Autodesk Fusion 360 part; units mm, degrees
(part 2 of 4)
  arc A354 (22.3833, -33.1693) -> (21.8833, -32.6693) centre (22.3833, -32.6693) cw
  arc A355 (35.3833, -19.1693) -> (35.8833, -19.6693) centre (35.3833, -19.6693) cw
  line L355 (21.8833, -32.6693) -> (21.8833, -19.6693)
  line L356 (35.8833, -0.6193) -> (35.8833, -13.6193)
  line L357 (21.8833, -13.6193) -> (21.8833, -0.6193)
  arc A356 (35.3833, -0.1193) -> (35.8833, -0.6193) centre (35.3833, -0.6193) cw
  arc A357 (35.8833, -13.6193) -> (35.3833, -14.1193) centre (35.3833, -13.6193) cw
  line L358 (22.3833, -0.1193) -> (35.3833, -0.1193)
  arc A358 (22.3833, -14.1193) -> (21.8833, -13.6193) centre (22.3833, -13.6193) cw
  line L359 (35.3833, -14.1193) -> (22.3833, -14.1193)
  arc A359 (21.8833, -0.6193) -> (22.3833, -0.1193) centre (22.3833, -0.6193) cw
  line L360 (22.3833, 18.9307) -> (35.3833, 18.9307)
  line L361 (35.3833, 4.9307) -> (22.3833, 4.9307)
  arc A360 (21.8833, 18.4307) -> (22.3833, 18.9307) centre (22.3833, 18.4307) cw
  arc A361 (35.8833, 5.4307) -> (35.3833, 4.9307) centre (35.3833, 5.4307) cw
  line L362 (21.8833, 5.4307) -> (21.8833, 18.4307)
  arc A362 (22.3833, 4.9307) -> (21.8833, 5.4307) centre (22.3833, 5.4307) cw
  arc A363 (35.3833, 18.9307) -> (35.8833, 18.4307) centre (35.3833, 18.4307) cw
  line L363 (35.8833, 18.4307) -> (35.8833, 5.4307)
  arc A364 (22.3833, 23.9807) -> (21.8833, 24.4807) centre (22.3833, 24.4807) cw
  arc A365 (35.3833, 37.9807) -> (35.8833, 37.4807) centre (35.3833, 37.4807) cw
  line L364 (35.8833, 37.4807) -> (35.8833, 24.4807)
  arc A366 (35.8833, 24.4807) -> (35.3833, 23.9807) centre (35.3833, 24.4807) cw
  line L365 (22.3833, 37.9807) -> (35.3833, 37.9807)
  arc A367 (21.8833, 37.4807) -> (22.3833, 37.9807) centre (22.3833, 37.4807) cw
  line L366 (35.3833, 23.9807) -> (22.3833, 23.9807)
  line L367 (21.8833, 24.4807) -> (21.8833, 37.4807)
  arc A368 (21.8833, 56.5307) -> (22.3833, 57.0307) centre (22.3833, 56.5307) cw
  arc A369 (22.3833, 43.0307) -> (21.8833, 43.5307) centre (22.3833, 43.5307) cw
  line L368 (22.3833, 57.0307) -> (35.3833, 57.0307)
  line L369 (35.3833, 43.0307) -> (22.3833, 43.0307)
  line L370 (21.8833, 43.5307) -> (21.8833, 56.5307)
  arc A370 (35.8833, 43.5307) -> (35.3833, 43.0307) centre (35.3833, 43.5307) cw
  arc A371 (35.3833, 57.0307) -> (35.8833, 56.5307) centre (35.3833, 56.5307) cw
  line L371 (35.8833, 56.5307) -> (35.8833, 43.5307)
  line L372 (22.3833, 76.0807) -> (35.3833, 76.0807)
  arc A372 (35.3833, 76.0807) -> (35.8833, 75.5807) centre (35.3833, 75.5807) cw
  arc A373 (35.8833, 62.5807) -> (35.3833, 62.0807) centre (35.3833, 62.5807) cw
  arc A374 (21.8833, 75.5807) -> (22.3833, 76.0807) centre (22.3833, 75.5807) cw
  line L373 (21.8833, 62.5807) -> (21.8833, 75.5807)
  line L374 (35.8833, 75.5807) -> (35.8833, 62.5807)
  line L375 (35.3833, 62.0807) -> (22.3833, 62.0807)
  arc A375 (22.3833, 62.0807) -> (21.8833, 62.5807) centre (22.3833, 62.5807) cw
  line L376 (22.3833, 95.1307) -> (35.3833, 95.1307)
  arc A376 (35.3833, 95.1307) -> (35.8833, 94.6307) centre (35.3833, 94.6307) cw
  line L377 (35.3833, 81.1307) -> (22.3833, 81.1307)
  line L378 (35.8833, 94.6307) -> (35.8833, 81.6307)
  arc A377 (35.8833, 81.6307) -> (35.3833, 81.1307) centre (35.3833, 81.6307) cw
  line L379 (21.8833, 81.6307) -> (21.8833, 94.6307)
  arc A378 (21.8833, 94.6307) -> (22.3833, 95.1307) centre (22.3833, 94.6307) cw
  arc A379 (22.3833, 81.1307) -> (21.8833, 81.6307) centre (22.3833, 81.6307) cw
  line L380 (35.3833, 116.8495) -> (22.3833, 116.8495)
  arc A380 (22.3833, 116.8495) -> (21.8833, 117.3495) centre (22.3833, 117.3495) cw
  arc A381 (35.8833, 117.3495) -> (35.3833, 116.8495) centre (35.3833, 117.3495) cw
  arc A382 (35.3833, 130.8495) -> (35.8833, 130.3495) centre (35.3833, 130.3495) cw
  line L381 (21.8833, 117.3495) -> (21.8833, 130.3495)
  arc A383 (21.8833, 130.3495) -> (22.3833, 130.8495) centre (22.3833, 130.3495) cw
  line L382 (35.8833, 130.3495) -> (35.8833, 117.3495)
  line L383 (22.3833, 130.8495) -> (35.3833, 130.8495)
  arc A384 (19.8833, 114.9115) -> (20.3833, 115.4115) centre (20.3833, 114.9115) cw
  arc A385 (34.8833, 108.9115) -> (34.3833, 108.4115) centre (34.3833, 108.9115) cw
  line L384 (20.3833, 115.4115) -> (34.3833, 115.4115)
  line L385 (34.3833, 108.4115) -> (20.3833, 108.4115)
  line L386 (34.8833, 114.9115) -> (34.8833, 108.9115)
  arc A386 (34.3833, 115.4115) -> (34.8833, 114.9115) centre (34.3833, 114.9115) cw
  line L387 (19.8833, 108.9115) -> (19.8833, 114.9115)
  arc A387 (20.3833, 108.4115) -> (19.8833, 108.9115) centre (20.3833, 108.9115) cw
  line L388 (19.8833, 132.7875) -> (19.8833, 138.7875)
  arc A388 (34.3833, 139.2875) -> (34.8833, 138.7875) centre (34.3833, 138.7875) cw
  line L389 (20.3833, 139.2875) -> (34.3833, 139.2875)
  line L390 (34.3833, 132.2875) -> (20.3833, 132.2875)
  line L391 (34.8833, 138.7875) -> (34.8833, 132.7875)
  arc A389 (19.8833, 138.7875) -> (20.3833, 139.2875) centre (20.3833, 138.7875) cw
  arc A390 (34.8833, 132.7875) -> (34.3833, 132.2875) centre (34.3833, 132.7875) cw
  arc A391 (20.3833, 132.2875) -> (19.8833, 132.7875) centre (20.3833, 132.7875) cw
  line L392 (35.8833, 194.6432) -> (35.8833, 181.6432)
  line L393 (22.3833, 195.1432) -> (35.3833, 195.1432)
  line L394 (35.3833, 181.1432) -> (22.3833, 181.1432)
  line L395 (21.8833, 181.6432) -> (21.8833, 194.6432)
  arc A392 (35.8833, 181.6432) -> (35.3833, 181.1432) centre (35.3833, 181.6432) cw
  arc A393 (35.3833, 195.1432) -> (35.8833, 194.6432) centre (35.3833, 194.6432) cw
  arc A394 (22.3833, 181.1432) -> (21.8833, 181.6432) centre (22.3833, 181.6432) cw
  arc A395 (21.8833, 194.6432) -> (22.3833, 195.1432) centre (22.3833, 194.6432) cw
  arc A396 (41.4333, -204.6193) -> (40.9332, -204.1193) centre (41.4333, -204.1193) cw
  line L396 (54.9333, -191.1193) -> (54.9332, -204.1193)
  line L397 (40.9332, -204.1193) -> (40.9333, -191.1193)
  arc A397 (40.9333, -191.1193) -> (41.4333, -190.6193) centre (41.4333, -191.1193) cw
  line L398 (41.4333, -190.6193) -> (54.4333, -190.6193)
  arc A398 (54.9332, -204.1193) -> (54.4332, -204.6193) centre (54.4333, -204.1193) cw
  line L399 (54.4332, -204.6193) -> (41.4333, -204.6193)
  arc A399 (54.4333, -190.6193) -> (54.9332, -191.1193) centre (54.4333, -191.1193) cw
  line L400 (41.4333, -162.0443) -> (54.4333, -162.0443)
  line L401 (54.9333, -162.5443) -> (54.9332, -175.5443)
  arc A400 (41.4333, -176.0443) -> (40.9333, -175.5443) centre (41.4333, -175.5443) cw
  arc A401 (54.9332, -175.5443) -> (54.4333, -176.0443) centre (54.4333, -175.5443) cw
  arc A402 (40.9333, -162.5443) -> (41.4333, -162.0443) centre (41.4333, -162.5443) cw
  line L402 (40.9333, -175.5443) -> (40.9333, -162.5443)
  arc A403 (54.4333, -162.0443) -> (54.9333, -162.5443) centre (54.4333, -162.5443) cw
  line L403 (54.4333, -176.0443) -> (41.4333, -176.0443)
  arc A404 (54.9333, -125.538) -> (54.4333, -126.038) centre (54.4333, -125.538) cw
  line L404 (41.4333, -112.038) -> (54.4333, -112.038)
  arc A405 (41.4333, -126.038) -> (40.9333, -125.538) centre (41.4333, -125.538) cw
  line L405 (54.4333, -126.038) -> (41.4333, -126.038)
  arc A406 (40.9333, -112.538) -> (41.4333, -112.038) centre (41.4333, -112.538) cw
  arc A407 (54.4333, -112.038) -> (54.9333, -112.538) centre (54.4333, -112.538) cw
  line L406 (54.9333, -112.538) -> (54.9333, -125.538)
  line L407 (40.9333, -125.538) -> (40.9333, -112.538)
  arc A408 (54.4333, -88.2255) -> (54.9333, -88.7255) centre (54.4333, -88.7255) cw
  arc A409 (41.4333, -102.2255) -> (40.9333, -101.7255) centre (41.4333, -101.7255) cw
  arc A410 (54.9333, -101.7255) -> (54.4333, -102.2255) centre (54.4333, -101.7255) cw
  line L408 (41.4333, -88.2255) -> (54.4333, -88.2255)
  arc A411 (40.9333, -88.7255) -> (41.4333, -88.2255) centre (41.4333, -88.7255) cw
  line L409 (54.9333, -88.7255) -> (54.9333, -101.7255)
  line L410 (40.9333, -101.7255) -> (40.9333, -88.7255)
  line L411 (54.4333, -102.2255) -> (41.4333, -102.2255)
  line L412 (54.9333, -64.913) -> (54.9333, -77.913)
  arc A412 (40.9333, -64.913) -> (41.4333, -64.413) centre (41.4333, -64.913) cw
  line L413 (41.4333, -64.413) -> (54.4333, -64.413)
  line L414 (40.9333, -77.913) -> (40.9333, -64.913)
  arc A413 (54.4333, -64.413) -> (54.9333, -64.913) centre (54.4333, -64.913) cw
  arc A414 (54.9333, -77.913) -> (54.4333, -78.413) centre (54.4333, -77.913) cw
  line L415 (54.4333, -78.413) -> (41.4333, -78.413)
  arc A415 (41.4333, -78.413) -> (40.9333, -77.913) centre (41.4333, -77.913) cw
  arc A416 (40.9333, 6.5245) -> (41.4333, 7.0245) centre (41.4333, 6.5245) cw
  line L416 (40.9333, -6.4755) -> (40.9333, 6.5245)
  line L417 (54.9333, 6.5245) -> (54.9333, -6.4755)
  arc A417 (54.4333, 7.0245) -> (54.9333, 6.5245) centre (54.4333, 6.5245) cw
  arc A418 (54.9333, -6.4755) -> (54.4333, -6.9755) centre (54.4333, -6.4755) cw
  arc A419 (41.4333, -6.9755) -> (40.9333, -6.4755) centre (41.4333, -6.4755) cw
  line L418 (41.4333, 7.0245) -> (54.4333, 7.0245)
  line L419 (54.4333, -6.9755) -> (41.4333, -6.9755)
  arc A420 (53.4333, -46.4755) -> (53.9333, -46.9755) centre (53.4333, -46.9755) cw
  line L420 (39.4333, -46.4755) -> (53.4333, -46.4755)
  arc A421 (39.4333, -53.4755) -> (38.9333, -52.9755) centre (39.4333, -52.9755) cw
  arc A422 (38.9332, -46.9755) -> (39.4333, -46.4755) centre (39.4333, -46.9755) cw
  line L421 (53.9333, -46.9755) -> (53.9333, -52.9755)
  arc A423 (53.9333, -52.9755) -> (53.4333, -53.4755) centre (53.4333, -52.9755) cw
  line L422 (53.4333, -53.4755) -> (39.4333, -53.4755)
  line L423 (38.9333, -52.9755) -> (38.9332, -46.9755)
  line L424 (38.9333, 47.0245) -> (38.9333, 53.0245)
  line L425 (53.4333, 46.5245) -> (39.4333, 46.5245)
  line L426 (39.4333, 53.5245) -> (53.4333, 53.5245)
  arc A424 (39.4333, 46.5245) -> (38.9333, 47.0245) centre (39.4333, 47.0245) cw
  arc A425 (53.4333, 53.5245) -> (53.9333, 53.0245) centre (53.4333, 53.0245) cw
  line L427 (53.9333, 53.0245) -> (53.9333, 47.0245)
  arc A426 (38.9333, 53.0245) -> (39.4333, 53.5245) centre (39.4333, 53.0245) cw
  arc A427 (53.9333, 47.0245) -> (53.4333, 46.5245) centre (53.4333, 47.0245) cw
  arc A428 (40.9333, 77.962) -> (41.4333, 78.462) centre (41.4333, 77.962) cw
  arc A429 (54.9333, 64.962) -> (54.4333, 64.462) centre (54.4333, 64.962) cw
  arc A430 (54.4333, 78.462) -> (54.9333, 77.962) centre (54.4333, 77.962) cw
  line L428 (40.9333, 64.962) -> (40.9333, 77.962)
  arc A431 (41.4333, 64.462) -> (40.9333, 64.962) centre (41.4333, 64.962) cw
  line L429 (54.4333, 64.462) -> (41.4333, 64.462)
  line L430 (54.9333, 77.962) -> (54.9333, 64.962)
  line L431 (41.4333, 78.462) -> (54.4333, 78.462)
  arc A432 (40.9333, 101.7745) -> (41.4333, 102.2745) centre (41.4333, 101.7745) cw
  line L432 (54.9333, 101.7745) -> (54.9333, 88.7745)
  arc A433 (54.4333, 102.2745) -> (54.9333, 101.7745) centre (54.4333, 101.7745) cw
  arc A434 (41.4333, 88.2745) -> (40.9333, 88.7745) centre (41.4333, 88.7745) cw
  line L433 (54.4333, 88.2745) -> (41.4333, 88.2745)
  line L434 (40.9333, 88.7745) -> (40.9333, 101.7745)
  line L435 (41.4333, 102.2745) -> (54.4333, 102.2745)
  arc A435 (54.9333, 88.7745) -> (54.4333, 88.2745) centre (54.4333, 88.7745) cw
  arc A436 (54.9333, 112.587) -> (54.4333, 112.087) centre (54.4333, 112.587) cw
  arc A437 (40.9332, 125.587) -> (41.4333, 126.087) centre (41.4333, 125.587) cw
  line L436 (54.4333, 112.087) -> (41.4333, 112.087)
  arc A438 (41.4333, 112.087) -> (40.9333, 112.587) centre (41.4333, 112.587) cw
  line L437 (40.9333, 112.587) -> (40.9332, 125.587)
  line L438 (41.4333, 126.087) -> (54.4333, 126.087)
  line L439 (54.9333, 125.587) -> (54.9333, 112.587)
  arc A439 (54.4333, 126.087) -> (54.9333, 125.587) centre (54.4333, 125.587) cw
  line L440 (54.9333, 147.0182) -> (54.9333, 134.0182)
  line L441 (41.4333, 147.5182) -> (54.4333, 147.5182)
  arc A440 (40.9333, 147.0182) -> (41.4333, 147.5182) centre (41.4333, 147.0182) cw
  arc A441 (54.9333, 134.0182) -> (54.4333, 133.5182) centre (54.4333, 134.0182) cw
  line L442 (40.9333, 134.0182) -> (40.9333, 147.0182)
  arc A442 (41.4333, 133.5182) -> (40.9333, 134.0182) centre (41.4333, 134.0182) cw
  line L443 (54.4333, 133.5182) -> (41.4333, 133.5182)
  arc A443 (54.4333, 147.5182) -> (54.9333, 147.0182) centre (54.4333, 147.0182) cw
  line L444 (41.4333, 176.0932) -> (54.4333, 176.0932)
  arc A444 (54.9333, 162.5932) -> (54.4333, 162.0932) centre (54.4333, 162.5932) cw
  line L445 (40.9333, 162.5932) -> (40.9333, 175.5932)
  arc A445 (41.4333, 162.0932) -> (40.9333, 162.5932) centre (41.4333, 162.5932) cw
  line L446 (54.4333, 162.0932) -> (41.4333, 162.0932)
  arc A446 (54.4333, 176.0932) -> (54.9333, 175.5932) centre (54.4333, 175.5932) cw
  line L447 (54.9333, 175.5932) -> (54.9333, 162.5932)
  arc A447 (40.9333, 175.5932) -> (41.4333, 176.0932) centre (41.4333, 175.5932) cw
  line L448 (41.4333, 195.1432) -> (54.4333, 195.1432)
  arc A448 (54.9333, 181.6432) -> (54.4333, 181.1432) centre (54.4333, 181.6432) cw
  line L449 (40.9333, 181.6432) -> (40.9333, 194.6432)
  line L450 (54.9333, 194.6432) -> (54.9333, 181.6432)
  arc A449 (41.4333, 181.1432) -> (40.9333, 181.6432) centre (41.4333, 181.6432) cw
  arc A450 (54.4333, 195.1432) -> (54.9333, 194.6432) centre (54.4333, 194.6432) cw
  line L451 (54.4333, 181.1432) -> (41.4333, 181.1432)
  arc A451 (40.9333, 194.6432) -> (41.4333, 195.1432) centre (41.4333, 194.6432) cw
  line L452 (40.9333, 200.6932) -> (40.9333, 213.6932)
  arc A452 (54.4333, 214.1932) -> (54.9333, 213.6932) centre (54.4333, 213.6932) cw
  arc A453 (41.4333, 200.1932) -> (40.9333, 200.6932) centre (41.4333, 200.6932) cw
  line L453 (41.4333, 214.1932) -> (54.4333, 214.1932)
  line L454 (54.9333, 213.6932) -> (54.9333, 200.6932)
  arc A454 (40.9333, 213.6932) -> (41.4333, 214.1932) centre (41.4333, 213.6932) cw
  line L455 (54.4333, 200.1932) -> (41.4333, 200.1932)
  arc A455 (54.9333, 200.6932) -> (54.4333, 200.1932) centre (54.4333, 200.6932) cw
  line L456 (58.3332, -216.6443) -> (58.3333, 224.1932)
  line L457 (-61.771, -216.6443) -> (-61.771, 224.1932)
  line L458 (58.3332, -216.6443) -> (-61.771, -216.6443)
  line L459 (58.3333, 224.1932) -> (-61.771, 224.1932)
  line L460 (58.3332, -216.6443) -> (-37.7668, -216.6443)
  line L461 (-37.7668, -216.6443) -> (-37.7667, -166.6443)
  line L462 (-37.7667, -166.6443) -> (-61.771, -166.6443)
  line L463 (-61.771, 150.0182) -> (-28.2417, 150.0182)
  line L464 (-28.2417, 150.0182) -> (-28.2417, 224.1932)
  line L465 (-28.2417, 224.1932) -> (58.3333, 224.1932)
  line L466 (-61.771, 150.0182) -> (-61.771, -166.6443) construction
  line L467 (63.4708, 230.5) -> (-67.5292, 230.5)
  line L468 (-67.5292, 230.5) -> (-67.5292, -230.5)
  line L469 (-67.5292, -230.5) -> (63.4708, -230.5)
  line L470 (63.4708, -230.5) -> (63.4708, 230.5)
  line L471 (-67.0292, -230) -> (62.9708, -230)
  line L472 (-66.7431, 215) -> (-32.0292, 215)
  line L473 (-66.7431, 150) -> (-66.7431, -166.6443)
  line L474 (-66.7431, -166.6443) -> (-37.7667, -166.6443)
  line L475 (-37.7667, -166.6443) -> (-37.7668, -230)
  line L476 (-66.7431, 230) -> (-66.7431, 215)
  line L477 (-37.7668, -230) -> (62.9708, -230)
  line L478 (62.9708, 230) -> (-66.7431, 230)
  line L479 (-32.0292, 215) -> (-32.0292, 150)
  line L480 (-32.0292, 150) -> (-66.7431, 150)
  line L481 (62.9708, -230) -> (62.9708, 230)
  line L482 (-66.7431, 150) -> (-66.7431, 230)
  line L483 (-66.7431, 230) -> (62.9708, 230)
  line L484 (62.9708, 230) -> (62.9708, 231.4)
  line L485 (62.9708, 231.4) -> (-66.7431, 231.4)
  line L486 (-66.7431, 231.4) -> (-66.7431, 230)
  line L487 (-37.7668, -230) -> (62.9708, -230)
  line L488 (62.9708, -230) -> (62.9708, -228.6)
  line L489 (62.9708, -228.6) -> (-37.7668, -228.6)
  line L490 (-37.7668, -228.6) -> (-37.7668, -230)
  line L491 (62.9708, -230) -> (61.7708, -230)
  line L492 (61.7708, -230) -> (61.7708, 231.4118)
  line L493 (61.7708, 231.4118) -> (62.9708, 231.4118)
  line L494 (62.9708, 231.4118) -> (62.9708, -230)
  line L495 (-66.7431, -166.6443) -> (-67.9431, -166.6443)
  line L496 (-67.9431, -166.6443) -> (-67.9431, 231.4)
  line L497 (-67.9431, 231.4) -> (-66.7431, 231.4)
  line L498 (-66.7431, 231.4) -> (-66.7431, -166.6443)
  line L499 (-67.9431, -166.6443) -> (-62.9431, -166.6443) construction
  line L500 (-62.9431, -166.6443) -> (-62.9431, -161.6443) construction
  line L501 (-62.9431, -161.6443) -> (-67.9431, -161.6443) construction
  line L502 (-67.9431, -161.6443) -> (-67.9431, -166.6443) construction
  circle A456 centre (-62.9431, -161.6443) radius 1.5
  line L503 (-62.9431, -161.6443) -> (-42.9431, -161.6443) construction
  circle A457 centre (-42.9431, -161.6443) radius 1.5
  line L504 (-37.7668, -228.6) -> (-27.4668, -228.6) construction
  line L505 (-27.4668, -228.6) -> (-27.4668, -224.6) construction
  line L506 (-27.4668, -224.6) -> (-37.7668, -224.6) construction
  line L507 (-37.7668, -224.6) -> (-37.7668, -228.6) construction
  circle A458 centre (-27.4668, -224.6) radius 1.7
  line L508 (61.7708, -228.6) -> (57.5708, -228.6)
  line L509 (57.5708, -228.6) -> (57.5708, -224.6) construction
  line L510 (57.5708, -224.6) -> (61.7708, -224.6) construction
  line L511 (61.7708, -224.6) -> (61.7708, -228.6)
  circle A459 centre (57.5708, -224.6) radius 1.7
  line L512 (61.7708, 231.4118) -> (57.1708, 231.4118) construction
  line L513 (57.1708, 231.4118) -> (57.1708, 227.4118) construction
  line L514 (57.1708, 227.4118) -> (61.7708, 227.4118) construction
  line L515 (61.7708, 227.4118) -> (61.7708, 231.4118) construction
  circle A460 centre (57.1708, 227.4118) radius 2
  line L516 (-67.9431, 231.4) -> (-63.3431, 231.4)
  line L517 (-63.3431, 231.4) -> (-63.3431, 227.4) construction
  line L518 (-63.3431, 227.4) -> (-67.9431, 227.4) construction
  line L519 (-67.9431, 227.4) -> (-67.9431, 231.4)
  circle A461 centre (-63.3431, 227.4) radius 2
  line L520 (-61.771, 169.5843) -> (-53.671, 169.5843) construction
  line L521 (-32.0292, 171.3559) -> (-39.7292, 171.3559) construction
  line L522 (-47.3464, 150.0182) -> (-47.3464, 161.0182) construction
  line L523 (-47.3464, 161.0182) -> (-47.3464, 185.8182) construction
  line L524 (-39.7292, 161.0182) -> (-53.671, 161.0182)
  line L525 (-53.671, 161.0182) -> (-53.671, 185.8182)
  line L526 (-53.671, 185.8182) -> (-39.7292, 185.8182)
  line L527 (-39.7292, 185.8182) -> (-39.7292, 161.0182)
  line L528 (-45.3649, 185.8182) -> (-45.3649, 194.2182) construction
  line L529 (-45.3649, 194.2182) -> (-45.3649, 207.2182) construction
  line L530 (-32.0292, 200.6083) -> (-40.6292, 200.6083) construction
  line L531 (-61.771, 201.3384) -> (-53.671, 201.3384) construction
  line L532 (-40.6292, 194.2182) -> (-53.671, 194.2182)
  line L533 (-53.671, 194.2182) -> (-53.671, 207.2182)
  line L534 (-53.671, 207.2182) -> (-40.6292, 207.2182)
  line L535 (-40.6292, 207.2182) -> (-40.6292, 194.2182)
  line L536 (-34.7292, 156.0182) -> (-58.671, 156.0182)
  line L537 (-58.671, 156.0182) -> (-58.671, 190.8182) construction
  line L538 (-58.671, 190.8182) -> (-34.7292, 190.8182)
  line L539 (-34.7292, 190.8182) -> (-34.7292, 156.0182) construction
  line L540 (-58.671, 190.8182) -> (-61.771, 190.8182)
  line L541 (-58.671, 156.0182) -> (-61.771, 156.0182)
  line L542 (-34.7292, 156.0182) -> (-32.0292, 156.0182)
  line L543 (-34.7292, 190.8182) -> (-32.0292, 190.8182)
  arc A462 (-34.2667, 124.9115) -> (-33.7667, 125.4115) centre (-33.7667, 124.9115) cw
  line L544 (-34.2667, 118.9115) -> (-34.2667, 124.9115)
  line L545 (-19.2667, 124.9115) -> (-19.2667, 118.9115)
  arc A463 (-19.7667, 125.4115) -> (-19.2667, 124.9115) centre (-19.7667, 124.9115) cw
  line L546 (-33.7667, 125.4115) -> (-19.7667, 125.4115)
  line L547 (-19.7667, 118.4115) -> (-33.7667, 118.4115)
  arc A464 (-19.2667, 118.9115) -> (-19.7667, 118.4115) centre (-19.7667, 118.9115) cw
  arc A465 (-33.7667, 118.4115) -> (-34.2667, 118.9115) centre (-33.7667, 118.9115) cw
  line L548 (-33.7667, 149.2875) -> (-19.7667, 149.2875)
  arc A466 (-34.2667, 148.7875) -> (-33.7667, 149.2875) centre (-33.7667, 148.7875) cw
  arc A467 (-19.7667, 149.2875) -> (-19.2667, 148.7875) centre (-19.7667, 148.7875) cw
  line L549 (-19.2667, 148.7875) -> (-19.2667, 142.7875)
  line L550 (-19.7667, 142.2875) -> (-33.7667, 142.2875)
  line L551 (-34.2667, 142.7875) -> (-34.2667, 148.7875)
  arc A468 (-19.2667, 142.7875) -> (-19.7667, 142.2875) centre (-19.7667, 142.7875) cw
  arc A469 (-33.7667, 142.2875) -> (-34.2667, 142.7875) centre (-33.7667, 142.7875) cw
  dimension "d3" = 1
  dimension "d4" = 2
  dimension "d5" = 14
  dimension "d6" = 6
  dimension "d7" = 1.4
  dimension "d8" = 1.4
  dimension "d9" = 1.2
  dimension "d10" = 1.2
  dimension "d14" = 5
  dimension "d15" = 5
  dimension "d16" = 3
  dimension "d17" = 20
  dimension "d18" = 3
  dimension "d22" = 10.3
  dimension "d23" = 4
  dimension "d24" = 3.4
  dimension "d25" = 4.2
  dimension "d26" = 4
  dimension "d27" = 3.4
  dimension "d28" = 4.6
  dimension "d29" = 4
  dimension "d30" = 4
  dimension "d31" = 4.6
  dimension "d32" = 4
  dimension "d33" = 4
  dimension "d34" = 8.1
  dimension "d35" = 7.7
  dimension "d36" = 11
  dimension "d37" = 24.8
  dimension "d38" = 8.4
  dimension "d39" = 13
  dimension "d40" = 8.6
  dimension "d41" = 8.1
  dimension "d42" = -5
  dimension "d116" = 1
  dimension "d117" = 1
  dimension "d118" = 2
  dimension "d119" = 2
  dimension "d120" = 1
  dimension "d121" = 1
  dimension "d122" = 2
  dimension "d123" = 2
  dimension "d124" = 1
  dimension "d125" = 1
  dimension "d126" = 2
  dimension "d127" = 2
  dimension "d128" = 16.876
  dimension "d129" = 1.438
  dimension "d130" = 1.438
  dimension "d131" = 2
  dimension "d132" = 2
  dimension "d133" = 1
  dimension "d134" = 1
  constraint equal L325 L327
  constraint equal L324 L326
  constraint vertical L325
  constraint horizontal L326
  constraint perpendicular L326 L327
  constraint perpendicular L324 L325
  constraint horizontal L483
  constraint vertical L484
  constraint horizontal L485
  constraint vertical L486
  constraint horizontal L487
  constraint vertical L488
  constraint horizontal L489
  constraint parallel L488 L490
  constraint horizontal L491
  constraint vertical L492
  constraint horizontal L493
  constraint vertical L494
  constraint horizontal L495
  constraint vertical L496
  constraint horizontal L497
  constraint vertical L498
  constraint horizontal L499
  constraint vertical L500
  constraint horizontal L501
  constraint vertical L502
  constraint coincident L500.end L501.start
  constraint perpendicular L457 L503
  constraint coincident L503.end A457.centre
  constraint vertical L505
  constraint perpendicular L504 L505
  constraint horizontal L506
  constraint parallel L505 L507
  constraint coincident L505.end L506.start
  constraint vertical L509
  constraint perpendicular L508 L509
  constraint horizontal L510
  constraint parallel L509 L511
  constraint coincident L489 L508.start
  constraint coincident L492 L508.start
  constraint coincident L509.end L510.start
  constraint vertical L513
  constraint perpendicular L512 L513
  constraint horizontal L514
  constraint parallel L513 L515
  constraint coincident L513.end L514.start
  constraint horizontal L516
  constraint vertical L517
  constraint horizontal L518
  constraint vertical L519
  constraint coincident L517.end L518.start
  constraint coincident L457 L520.start
  constraint perpendicular L457 L520
  constraint coincident L479 L521.start
  constraint perpendicular L479 L521
  constraint coincident L463 L522.start
  constraint perpendicular L463 L522
  constraint parallel L522 L523
  constraint horizontal L524
  constraint vertical L525
  constraint horizontal L526
  constraint vertical L527
  constraint coincident L522.end L524
  constraint coincident L521.end L527
  constraint coincident L520.end L525
  constraint coincident L523.end L526
  constraint coincident L526 L528.start
  constraint perpendicular L526 L528
  constraint vertical L529
  constraint coincident L479 L530.start
  constraint perpendicular L479 L530
  constraint coincident L457 L531.start
  constraint perpendicular L457 L531
  constraint horizontal L532
  constraint vertical L533
  constraint horizontal L534
  constraint vertical L535
  constraint coincident L528.end L532
  constraint coincident L530.end L535
  constraint coincident L529.end L534
  constraint coincident L531.end L533
  constraint coincident L457 L540.end
  constraint perpendicular L457 L540
  constraint coincident L457 L541.end
  constraint perpendicular L457 L541
  constraint coincident L479 L542.end
  constraint perpendicular L479 L542
  constraint coincident L479 L543.end
  constraint perpendicular L479 L543
  measures "d3" distance of L329 L332
  measures "d4" distance of L331 L335
  measures "d5" distance of A325.end L325.end
  measures "d6" distance of A324.start L326.start
  measures "d7" distance of L476.start L485.end
  measures "d8" distance of L475.end L489.end
  measures "d9" distance of L471.end L491.end
  measures "d10" distance of L473.end L495.end
  measures "d14" distance of L495.end L499.end
  measures "d15" distance of L495.end L501.end
  measures "d16" diameter of A456
  measures "d17" distance of L500.end L503.end
  measures "d18" diameter of A457
  measures "d22" distance of L489.end L504.end
  measures "d23" distance of L489.end L506.end
  measures "d24" diameter of A458
  measures "d25" distance of L508.start L508.end
  measures "d26" distance of L508.start L510.end
  measures "d27" diameter of A459
  measures "d28" distance of L492.end L512.end
  measures "d29" distance of L492.end L514.end
  measures "d30" diameter of A460
  measures "d31" distance of L496.end L516.end
  measures "d32" distance of L496.end L518.end
  measures "d33" diameter of A461
  measures "d34" distance of L520.start L520.end
  measures "d35" distance of L521.start L521.end
  measures "d36" distance of L522.start L522.end
  measures "d37" distance of L522.end L523.end
  measures "d38" distance of L528.start L528.end
  measures "d39" distance of L528.end L529.end
  measures "d40" distance of L530.start L530.end
  measures "d41" distance of L531.start L531.end
  measures "d116" distance of L417 L421
  measures "d117" distance of L417 L427
  measures "d118" distance of L416 L423
  measures "d119" distance of L416 L424
  measures "d120" distance of L155 L161
  measures "d121" distance of L155 L158
  measures "d122" distance of L152 L157
  measures "d123" distance of L152 L163
  measures "d124" distance of L319 L320
  measures "d125" distance of L319 L324
  measures "d126" distance of L318 L322
  measures "d127" distance of L318 L326
  measures "d128" distance of L546 L550
  measures "d129" distance of L124 L550
  measures "d130" distance of L127 L546
  measures "d131" distance of L125 L545
  measures "d132" distance of L125 L549
  measures "d133" distance of L126 L551
  measures "d134" distance of L126 L544
extrude "Extrude1" add sketch "IronHandPCBPlate" along normal blind 2 contours L456 L457 L458 L459 L460 L461 L462 L463 L464 L465 L474 L475 L479 L480 A456 | L456 L457 L458 L459 L460 L465 L472 L475 L476 L478 L482 L483 L489 L492 L498 L508 L511 | L457 L459 L463 L464 L472 L479 | L457 L473 L474 L480 L498 A456 | L457 L472 L479 L538 L540 L543 | L457 L472 L480 L482 L498 | L457 L463 L479 L480 | L457 L463 L479 L536 L541 L542 | L467 L468 L473 L476 L482 L486 L495 L498 | L457 L479 L536 L538 L540 L541 L542 L543 | L467 L468 L486 L495 L496 L497 L498 L516 L519 | L467 L478 L483 L486 L492 L498 | L467 L485 L486 L492 L498 L516 makes body 1
sketch "Sketch3" plane through (0, 0, 2) normal (0, 0, 1) x (-1, 0, 0)
  arc A0 (35.2667, -62.5807) -> (34.7667, -62.0807) centre (34.7667, -62.5807) ccw
  line L0 (35.2667, -62.5807) -> (35.2667, -75.5807)
  arc A1 (34.7667, -76.0807) -> (35.2667, -75.5807) centre (34.7667, -75.5807) ccw
  line L1 (34.7667, -76.0807) -> (21.7667, -76.0807)
  arc A2 (21.2667, -75.5807) -> (21.7667, -76.0807) centre (21.7667, -75.5807) ccw
  line L2 (21.2667, -75.5807) -> (21.2667, -62.5807)
  arc A3 (21.7667, -62.0807) -> (21.2667, -62.5807) centre (21.7667, -62.5807) ccw
  line L3 (21.7667, -62.0807) -> (34.7667, -62.0807)
  circle A4 centre (62.9431, 161.6443) radius 1.5
  line L4 (-35.3833, 176.0443) -> (-22.3833, 176.0443)
  arc A5 (-21.8833, 175.5443) -> (-22.3833, 176.0443) centre (-22.3832, 175.5443) ccw
  line L5 (-21.8833, 175.5443) -> (-21.8833, 162.5443)
  arc A6 (-22.3833, 162.0443) -> (-21.8833, 162.5443) centre (-22.3833, 162.5443) ccw
  line L6 (-22.3833, 162.0443) -> (-35.3833, 162.0443)
  arc A7 (-35.8833, 162.5443) -> (-35.3833, 162.0443) centre (-35.3833, 162.5443) ccw
  line L7 (-35.8833, 162.5443) -> (-35.8833, 175.5443)
  arc A8 (-35.3833, 176.0443) -> (-35.8833, 175.5443) centre (-35.3833, 175.5443) ccw
  line L8 (-40.9333, -181.6432) -> (-40.9333, -194.6432)
  arc A9 (-41.4333, -195.1432) -> (-40.9333, -194.6432) centre (-41.4333, -194.6432) ccw
  line L9 (-41.4333, -195.1432) -> (-54.4333, -195.1432)
  arc A10 (-54.9333, -194.6432) -> (-54.4333, -195.1432) centre (-54.4333, -194.6432) ccw
  line L10 (-54.9333, -194.6432) -> (-54.9333, -181.6432)
  arc A11 (-54.4333, -181.1432) -> (-54.9333, -181.6432) centre (-54.4333, -181.6432) ccw
  line L11 (-54.4333, -181.1432) -> (-41.4333, -181.1432)
  arc A12 (-40.9333, -181.6432) -> (-41.4333, -181.1432) centre (-41.4333, -181.6432) ccw
  arc A13 (34.7667, 95.3693) -> (35.2667, 95.8693) centre (34.7667, 95.8693) ccw
  line L12 (34.7667, 95.3693) -> (21.7667, 95.3693)
  arc A14 (21.2667, 95.8693) -> (21.7667, 95.3693) centre (21.7667, 95.8693) ccw
  line L13 (21.2667, 95.8693) -> (21.2668, 108.8693)
  arc A15 (21.7667, 109.3693) -> (21.2667, 108.8693) centre (21.7667, 108.8693) ccw
  line L14 (21.7667, 109.3693) -> (34.7667, 109.3693)
  arc A16 (35.2668, 108.8693) -> (34.7667, 109.3693) centre (34.7667, 108.8693) ccw
  line L15 (35.2668, 108.8693) -> (35.2667, 95.8693)
  arc A17 (-54.4333, 176.0443) -> (-54.9333, 175.5443) centre (-54.4333, 175.5443) ccw
  line L16 (-54.4333, 176.0443) -> (-41.4333, 176.0443)
  arc A18 (-40.9333, 175.5443) -> (-41.4333, 176.0443) centre (-41.4332, 175.5443) ccw
  line L17 (-40.9333, 175.5443) -> (-40.9333, 162.5443)
  arc A19 (-41.4333, 162.0443) -> (-40.9333, 162.5443) centre (-41.4333, 162.5443) ccw
  line L18 (-41.4333, 162.0443) -> (-54.4333, 162.0443)
  arc A20 (-54.9333, 162.5443) -> (-54.4333, 162.0443) centre (-54.4333, 162.5443) ccw
  line L19 (-54.9333, 162.5443) -> (-54.9333, 175.5443)
  arc A21 (15.7167, 52.5068) -> (16.2167, 53.0068) centre (15.7167, 53.0068) ccw
  line L20 (15.7167, 52.5068) -> (2.7167, 52.5068)
  arc A22 (2.2167, 53.0068) -> (2.7167, 52.5068) centre (2.7167, 53.0068) ccw
  line L21 (2.2167, 53.0068) -> (2.2167, 66.0068)
  arc A23 (2.7167, 66.5068) -> (2.2167, 66.0068) centre (2.7167, 66.0068) ccw
  line L22 (2.7167, 66.5068) -> (15.7167, 66.5068)
  arc A24 (16.2167, 66.0068) -> (15.7167, 66.5068) centre (15.7167, 66.0068) ccw
  line L23 (16.2167, 66.0068) -> (16.2167, 53.0068)
  arc A25 (-38.9333, 52.9755) -> (-39.4333, 53.4755) centre (-39.4333, 52.9755) ccw
  line L24 (-38.9333, 52.9755) -> (-38.9332, 46.9755)
  arc A26 (-39.4333, 46.4755) -> (-38.9332, 46.9755) centre (-39.4333, 46.9755) ccw
  line L25 (-39.4333, 46.4755) -> (-53.4333, 46.4755)
  arc A27 (-53.9333, 46.9755) -> (-53.4333, 46.4755) centre (-53.4333, 46.9755) ccw
  line L26 (-53.9333, 46.9755) -> (-53.9333, 52.9755)
  arc A28 (-53.4333, 53.4755) -> (-53.9333, 52.9755) centre (-53.4333, 52.9755) ccw
  line L27 (-53.4333, 53.4755) -> (-39.4333, 53.4755)
  line L28 (-34.3833, -108.4115) -> (-20.3833, -108.4115)
  arc A29 (-19.8833, -108.9115) -> (-20.3833, -108.4115) centre (-20.3833, -108.9115) ccw
  line L29 (-19.8833, -108.9115) -> (-19.8833, -114.9115)
  arc A30 (-20.3833, -115.4115) -> (-19.8833, -114.9115) centre (-20.3833, -114.9115) ccw
  line L30 (-20.3833, -115.4115) -> (-34.3833, -115.4115)
  arc A31 (-34.8833, -114.9115) -> (-34.3833, -115.4115) centre (-34.3833, -114.9115) ccw
  line L31 (-34.8833, -114.9115) -> (-34.8833, -108.9115)
  arc A32 (-34.3833, -108.4115) -> (-34.8833, -108.9115) centre (-34.3833, -108.9115) ccw
  line L32 (34.7667, 142.9943) -> (21.7667, 142.9943)
  arc A33 (21.2668, 143.4943) -> (21.7667, 142.9943) centre (21.7667, 143.4943) ccw
  line L33 (21.2668, 143.4943) -> (21.2667, 156.4943)
  arc A34 (21.7667, 156.9943) -> (21.2667, 156.4943) centre (21.7667, 156.4943) ccw
  line L34 (21.7667, 156.9943) -> (34.7667, 156.9943)
  arc A35 (35.2667, 156.4943) -> (34.7667, 156.9943) centre (34.7667, 156.4943) ccw
  line L35 (35.2667, 156.4943) -> (35.2667, 143.4943)
  arc A36 (34.7667, 142.9943) -> (35.2667, 143.4943) centre (34.7667, 143.4943) ccw
  line L36 (-21.8833, 13.6193) -> (-21.8833, 0.6193)
  arc A37 (-22.3833, 0.1193) -> (-21.8833, 0.6193) centre (-22.3833, 0.6193) ccw
  line L37 (-22.3833, 0.1193) -> (-35.3833, 0.1193)
  arc A38 (-35.8833, 0.6193) -> (-35.3833, 0.1193) centre (-35.3833, 0.6193) ccw
  line L38 (-35.8833, 0.6193) -> (-35.8833, 13.6193)
  arc A39 (-35.3833, 14.1193) -> (-35.8833, 13.6193) centre (-35.3833, 13.6193) ccw
  line L39 (-35.3833, 14.1193) -> (-22.3833, 14.1193)
  arc A40 (-21.8833, 13.6193) -> (-22.3833, 14.1193) centre (-22.3833, 13.6193) ccw
  line L40 (58.5792, -90.3682) -> (45.5792, -90.3682)
  arc A41 (45.0792, -89.8682) -> (45.5792, -90.3682) centre (45.5792, -89.8682) ccw
  line L41 (45.0792, -89.8682) -> (45.0792, -76.8682)
  arc A42 (45.5792, -76.3682) -> (45.0792, -76.8682) centre (45.5792, -76.8682) ccw
  line L42 (45.5792, -76.3682) -> (58.5792, -76.3682)
  arc A43 (59.0792, -76.8682) -> (58.5792, -76.3682) centre (58.5792, -76.8682) ccw
  line L43 (59.0792, -76.8682) -> (59.0792, -89.8682)
  arc A44 (58.5792, -90.3682) -> (59.0792, -89.8682) centre (58.5792, -89.8682) ccw
  arc A45 (35.2667, -81.6307) -> (34.7667, -81.1307) centre (34.7667, -81.6307) ccw
  line L44 (35.2667, -81.6307) -> (35.2667, -94.6307)
  arc A46 (34.7667, -95.1307) -> (35.2667, -94.6307) centre (34.7667, -94.6307) ccw
  line L45 (34.7667, -95.1307) -> (21.7667, -95.1307)
  arc A47 (21.2667, -94.6307) -> (21.7667, -95.1307) centre (21.7667, -94.6307) ccw
  line L46 (21.2667, -94.6307) -> (21.2667, -81.6307)
  arc A48 (21.7667, -81.1307) -> (21.2667, -81.6307) centre (21.7667, -81.6307) ccw
  line L47 (21.7667, -81.1307) -> (34.7667, -81.1307)
  arc A49 (35.2667, 51.7193) -> (34.7667, 52.2193) centre (34.7667, 51.7193) ccw
  line L48 (35.2667, 51.7193) -> (35.2667, 38.7193)
  arc A50 (34.7667, 38.2193) -> (35.2667, 38.7193) centre (34.7667, 38.7193) ccw
  line L49 (34.7667, 38.2193) -> (21.7667, 38.2193)
  arc A51 (21.2667, 38.7193) -> (21.7667, 38.2193) centre (21.7667, 38.7193) ccw
  line L50 (21.2667, 38.7193) -> (21.2667, 51.7193)
  arc A52 (21.7667, 52.2193) -> (21.2667, 51.7193) centre (21.7667, 51.7193) ccw
  line L51 (21.7667, 52.2193) -> (34.7667, 52.2193)
  line L52 (-41.4333, -147.5182) -> (-54.4333, -147.5182)
  arc A53 (-54.9333, -147.0182) -> (-54.4333, -147.5182) centre (-54.4333, -147.0182) ccw
  line L53 (-54.9333, -147.0182) -> (-54.9333, -134.0182)
  arc A54 (-54.4333, -133.5182) -> (-54.9333, -134.0182) centre (-54.4333, -134.0182) ccw
  line L54 (-54.4333, -133.5182) -> (-41.4333, -133.5182)
  arc A55 (-40.9333, -134.0182) -> (-41.4333, -133.5182) centre (-41.4333, -134.0182) ccw
  line L55 (-40.9333, -134.0182) -> (-40.9333, -147.0182)
  arc A56 (-41.4333, -147.5182) -> (-40.9333, -147.0182) centre (-41.4333, -147.0182) ccw
  line L56 (21.7667, -4.9307) -> (34.7667, -4.9307)
  arc A57 (35.2667, -5.4307) -> (34.7667, -4.9307) centre (34.7667, -5.4307) ccw
  line L57 (35.2667, -5.4307) -> (35.2667, -18.4307)
  arc A58 (34.7667, -18.9307) -> (35.2667, -18.4307) centre (34.7667, -18.4307) ccw
  line L58 (34.7667, -18.9307) -> (21.7667, -18.9307)
  arc A59 (21.2667, -18.4307) -> (21.7667, -18.9307) centre (21.7667, -18.4307) ccw
  line L59 (21.2667, -18.4307) -> (21.2667, -5.4307)
  arc A60 (21.7667, -4.9307) -> (21.2667, -5.4307) centre (21.7667, -5.4307) ccw
  arc A61 (-2.8333, -14.9557) -> (-3.3333, -14.4557) centre (-3.3333, -14.9557) ccw
  line L60 (-2.8333, -14.9557) -> (-2.8333, -27.9557)
  arc A62 (-3.3333, -28.4557) -> (-2.8333, -27.9557) centre (-3.3333, -27.9557) ccw
  line L61 (-3.3333, -28.4557) -> (-16.3333, -28.4557)
  arc A63 (-16.8333, -27.9557) -> (-16.3333, -28.4557) centre (-16.3333, -27.9557) ccw
  line L62 (-16.8333, -27.9557) -> (-16.8333, -14.9557)
  arc A64 (-16.3333, -14.4557) -> (-16.8333, -14.9557) centre (-16.3333, -14.9557) ccw
  line L63 (-16.3333, -14.4557) -> (-3.3333, -14.4557)
  arc A65 (-16.8333, 181.5943) -> (-16.3333, 181.0943) centre (-16.3333, 181.5943) ccw
  line L64 (-16.8333, 181.5943) -> (-16.8333, 194.5943)
  arc A66 (-16.3333, 195.0943) -> (-16.8333, 194.5943) centre (-16.3333, 194.5943) ccw
  line L65 (-16.3333, 195.0943) -> (-3.3332, 195.0943)
  arc A67 (-2.8333, 194.5943) -> (-3.3332, 195.0943) centre (-3.3332, 194.5943) ccw
  line L66 (-2.8333, 194.5943) -> (-2.8332, 181.5943)
  arc A68 (-3.3332, 181.0943) -> (-2.8332, 181.5943) centre (-3.3333, 181.5943) ccw
  line L67 (-3.3332, 181.0943) -> (-16.3333, 181.0943)
  line L68 (2.2167, -80.3432) -> (2.2167, -67.3432)
  arc A69 (2.7167, -66.8432) -> (2.2167, -67.3432) centre (2.7167, -67.3432) ccw
  line L69 (2.7167, -66.8432) -> (15.7167, -66.8432)
  arc A70 (16.2167, -67.3432) -> (15.7167, -66.8432) centre (15.7167, -67.3432) ccw
  line L70 (16.2167, -67.3432) -> (16.2167, -80.3432)
  arc A71 (15.7167, -80.8432) -> (16.2167, -80.3432) centre (15.7167, -80.3432) ccw
  line L71 (15.7167, -80.8432) -> (2.7167, -80.8432)
  arc A72 (2.2167, -80.3432) -> (2.7167, -80.8432) centre (2.7167, -80.3432) ccw
  arc A73 (45.5792, -133.5182) -> (45.0792, -134.0182) centre (45.5792, -134.0182) ccw
  line L72 (45.5792, -133.5182) -> (58.5792, -133.5182)
  arc A74 (59.0792, -134.0182) -> (58.5792, -133.5182) centre (58.5792, -134.0182) ccw
  line L73 (59.0792, -134.0182) -> (59.0793, -147.0182)
  arc A75 (58.5792, -147.5182) -> (59.0793, -147.0182) centre (58.5792, -147.0182) ccw
  line L74 (58.5792, -147.5182) -> (45.5792, -147.5182)
  arc A76 (45.0792, -147.0182) -> (45.5792, -147.5182) centre (45.5792, -147.0182) ccw
  line L75 (45.0792, -147.0182) -> (45.0792, -134.0182)
  arc A77 (-35.8833, -18.4307) -> (-35.3833, -18.9307) centre (-35.3833, -18.4307) ccw
  line L76 (-35.8833, -18.4307) -> (-35.8833, -5.4307)
  arc A78 (-35.3833, -4.9307) -> (-35.8833, -5.4307) centre (-35.3833, -5.4307) ccw
  line L77 (-35.3833, -4.9307) -> (-22.3833, -4.9307)
  arc A79 (-21.8833, -5.4307) -> (-22.3833, -4.9307) centre (-22.3833, -5.4307) ccw
  line L78 (-21.8833, -5.4307) -> (-21.8833, -18.4307)
  arc A80 (-22.3833, -18.9307) -> (-21.8833, -18.4307) centre (-22.3833, -18.4307) ccw
  line L79 (-22.3833, -18.9307) -> (-35.3833, -18.9307)
  arc A81 (6.6917, -131.637) -> (6.1917, -131.137) centre (6.1917, -131.637) ccw
  line L80 (6.6917, -131.637) -> (6.6917, -144.637)
  arc A82 (6.1917, -145.137) -> (6.6917, -144.637) centre (6.1917, -144.637) ccw
  line L81 (6.1917, -145.137) -> (-6.8083, -145.137)
  arc A83 (-7.3083, -144.637) -> (-6.8083, -145.137) centre (-6.8083, -144.637) ccw
  line L82 (-7.3083, -144.637) -> (-7.3083, -131.637)
  arc A84 (-6.8083, -131.137) -> (-7.3083, -131.637) centre (-6.8083, -131.637) ccw
  line L83 (-6.8083, -131.137) -> (6.1917, -131.137)
  line L84 (-6.8083, -200.1932) -> (6.1917, -200.1932)
  arc A85 (6.6917, -200.6932) -> (6.1917, -200.1932) centre (6.1917, -200.6932) ccw
  line L85 (6.6917, -200.6932) -> (6.6917, -213.6932)
  arc A86 (6.1917, -214.1932) -> (6.6917, -213.6932) centre (6.1917, -213.6932) ccw
  line L86 (6.1917, -214.1932) -> (-6.8083, -214.1932)
  arc A87 (-7.3083, -213.6932) -> (-6.8083, -214.1932) centre (-6.8083, -213.6932) ccw
  line L87 (-7.3083, -213.6932) -> (-7.3083, -200.6932)
  arc A88 (-6.8083, -200.1932) -> (-7.3083, -200.6932) centre (-6.8083, -200.6932) ccw
  line L88 (-22.3833, 76.3193) -> (-35.3833, 76.3193)
  arc A89 (-35.8833, 76.8193) -> (-35.3833, 76.3193) centre (-35.3833, 76.8193) ccw
  line L89 (-35.8833, 76.8193) -> (-35.8833, 89.8193)
  arc A90 (-35.3833, 90.3193) -> (-35.8833, 89.8193) centre (-35.3833, 89.8193) ccw
  line L90 (-35.3833, 90.3193) -> (-22.3833, 90.3193)
  arc A91 (-21.8833, 89.8193) -> (-22.3833, 90.3193) centre (-22.3833, 89.8193) ccw
  line L91 (-21.8833, 89.8193) -> (-21.8833, 76.8193)
  arc A92 (-22.3833, 76.3193) -> (-21.8833, 76.8193) centre (-22.3833, 76.8193) ccw
  arc A93 (-54.4333, 6.9755) -> (-54.9333, 6.4755) centre (-54.4333, 6.4755) ccw
  line L92 (-54.4333, 6.9755) -> (-41.4333, 6.9755)
  arc A94 (-40.9333, 6.4755) -> (-41.4333, 6.9755) centre (-41.4333, 6.4755) ccw
  line L93 (-40.9333, 6.4755) -> (-40.9333, -6.5245)
  arc A95 (-41.4333, -7.0245) -> (-40.9333, -6.5245) centre (-41.4333, -6.5245) ccw
  line L94 (-41.4333, -7.0245) -> (-54.4333, -7.0245)
  arc A96 (-54.9333, -6.5245) -> (-54.4333, -7.0245) centre (-54.4333, -6.5245) ccw
  line L95 (-54.9333, -6.5245) -> (-54.9333, 6.4755)
  line L96 (59.0792, 127.9193) -> (59.0793, 114.9193)
  arc A97 (58.5792, 114.4193) -> (59.0793, 114.9193) centre (58.5793, 114.9193) ccw
  line L97 (58.5792, 114.4193) -> (45.5792, 114.4193)
  arc A98 (45.0793, 114.9193) -> (45.5792, 114.4193) centre (45.5793, 114.9193) ccw
  line L98 (45.0793, 114.9193) -> (45.0793, 127.9193)
  arc A99 (45.5792, 128.4193) -> (45.0793, 127.9193) centre (45.5792, 127.9193) ccw
  line L99 (45.5792, 128.4193) -> (58.5792, 128.4193)
  arc A100 (59.0792, 127.9193) -> (58.5792, 128.4193) centre (58.5792, 127.9193) ccw
  arc A101 (15.7167, -4.6432) -> (16.2167, -4.1432) centre (15.7167, -4.1432) ccw
  line L100 (15.7167, -4.6432) -> (2.7167, -4.6432)
  arc A102 (2.2167, -4.1432) -> (2.7167, -4.6432) centre (2.7167, -4.1432) ccw
  line L101 (2.2167, -4.1432) -> (2.2167, 8.8568)
  arc A103 (2.7167, 9.3568) -> (2.2167, 8.8568) centre (2.7167, 8.8568) ccw
  line L102 (2.7167, 9.3568) -> (15.7167, 9.3568)
  arc A104 (16.2167, 8.8568) -> (15.7167, 9.3568) centre (15.7167, 8.8568) ccw
  line L103 (16.2167, 8.8568) -> (16.2167, -4.1432)
  arc A105 (21.2668, 114.9193) -> (21.7667, 114.4193) centre (21.7667, 114.9193) ccw
  line L104 (21.2668, 114.9193) -> (21.2667, 127.9193)
  arc A106 (21.7667, 128.4193) -> (21.2667, 127.9193) centre (21.7667, 127.9193) ccw
  line L105 (21.7667, 128.4193) -> (34.7667, 128.4193)
  arc A107 (35.2667, 127.9193) -> (34.7667, 128.4193) centre (34.7667, 127.9193) ccw
  line L106 (35.2667, 127.9193) -> (35.2668, 114.9193)
  arc A108 (34.7667, 114.4193) -> (35.2668, 114.9193) centre (34.7667, 114.9193) ccw
  line L107 (34.7667, 114.4193) -> (21.7667, 114.4193)
  arc A109 (-3.3332, 200.1443) -> (-2.8332, 200.6443) centre (-3.3332, 200.6443) ccw
  line L108 (-3.3332, 200.1443) -> (-16.3333, 200.1443)
  arc A110 (-16.8333, 200.6443) -> (-16.3333, 200.1443) centre (-16.3333, 200.6443) ccw
  line L109 (-16.8333, 200.6443) -> (-16.8332, 213.6443)
  arc A111 (-16.3333, 214.1443) -> (-16.8333, 213.6443) centre (-16.3332, 213.6443) ccw
  line L110 (-16.3333, 214.1443) -> (-3.3332, 214.1443)
  arc A112 (-2.8332, 213.6443) -> (-3.3332, 214.1443) centre (-3.3333, 213.6443) ccw
  line L111 (-2.8332, 213.6443) -> (-2.8332, 200.6443)
  arc A113 (-22.3833, 200.1443) -> (-21.8832, 200.6443) centre (-22.3832, 200.6443) ccw
  line L112 (-22.3833, 200.1443) -> (-35.3833, 200.1443)
  arc A114 (-35.8833, 200.6443) -> (-35.3833, 200.1443) centre (-35.3833, 200.6443) ccw
  line L113 (-35.8833, 200.6443) -> (-35.8833, 213.6443)
  arc A115 (-35.3833, 214.1443) -> (-35.8833, 213.6443) centre (-35.3832, 213.6443) ccw
  line L114 (-35.3833, 214.1443) -> (-22.3832, 214.1443)
  arc A116 (-21.8833, 213.6443) -> (-22.3832, 214.1443) centre (-22.3832, 213.6443) ccw
  line L115 (-21.8833, 213.6443) -> (-21.8832, 200.6443)
  line L116 (-2.8333, 80.2943) -> (-2.8333, 67.2943)
  arc A117 (-3.3333, 66.7943) -> (-2.8333, 67.2943) centre (-3.3333, 67.2943) ccw
  line L117 (-3.3333, 66.7943) -> (-16.3333, 66.7943)
  arc A118 (-16.8333, 67.2943) -> (-16.3333, 66.7943) centre (-16.3333, 67.2943) ccw
  line L118 (-16.8333, 67.2943) -> (-16.8333, 80.2943)
  arc A119 (-16.3333, 80.7943) -> (-16.8333, 80.2943) centre (-16.3333, 80.2943) ccw
  line L119 (-16.3333, 80.7943) -> (-3.3333, 80.7943)
  arc A120 (-2.8333, 80.2943) -> (-3.3333, 80.7943) centre (-3.3333, 80.2943) ccw
  arc A121 (6.1917, -195.1432) -> (6.6917, -194.6432) centre (6.1917, -194.6432) ccw
  line L120 (6.1917, -195.1432) -> (-6.8083, -195.1432)
  arc A122 (-7.3083, -194.6432) -> (-6.8083, -195.1432) centre (-6.8083, -194.6432) ccw
  line L121 (-7.3083, -194.6432) -> (-7.3083, -181.6432)
  arc A123 (-6.8083, -181.1432) -> (-7.3083, -181.6432) centre (-6.8083, -181.6432) ccw
  line L122 (-6.8083, -181.1432) -> (6.1917, -181.1432)
  arc A124 (6.6917, -181.6432) -> (6.1917, -181.1432) centre (6.1917, -181.6432) ccw
  line L123 (6.6917, -181.6432) -> (6.6917, -194.6432)
  arc A125 (21.2667, 162.5443) -> (21.7667, 162.0443) centre (21.7667, 162.5443) ccw
  line L124 (21.2667, 162.5443) -> (21.2667, 175.5443)
  arc A126 (21.7667, 176.0443) -> (21.2667, 175.5443) centre (21.7667, 175.5443) ccw
  line L125 (21.7667, 176.0443) -> (34.7667, 176.0443)
  arc A127 (35.2668, 175.5443) -> (34.7667, 176.0443) centre (34.7667, 175.5443) ccw
  line L126 (35.2668, 175.5443) -> (35.2667, 162.5443)
  arc A128 (34.7667, 162.0443) -> (35.2668, 162.5443) centre (34.7667, 162.5443) ccw
  line L127 (34.7667, 162.0443) -> (21.7667, 162.0443)
  line L128 (-54.9333, -213.6932) -> (-54.9333, -200.6932)
  arc A129 (-54.4333, -200.1932) -> (-54.9333, -200.6932) centre (-54.4333, -200.6932) ccw
  line L129 (-54.4333, -200.1932) -> (-41.4333, -200.1932)
  arc A130 (-40.9333, -200.6932) -> (-41.4333, -200.1932) centre (-41.4333, -200.6932) ccw
  line L130 (-40.9333, -200.6932) -> (-40.9333, -213.6932)
  arc A131 (-41.4333, -214.1932) -> (-40.9333, -213.6932) centre (-41.4333, -213.6932) ccw
  line L131 (-41.4333, -214.1932) -> (-54.4333, -214.1932)
  arc A132 (-54.9333, -213.6932) -> (-54.4333, -214.1932) centre (-54.4333, -213.6932) ccw
  arc A133 (8.1297, -146.637) -> (8.6297, -147.137) centre (8.6297, -146.637) ccw
  line L132 (8.1297, -146.637) -> (8.1297, -132.637)
  arc A134 (8.6297, -132.137) -> (8.1297, -132.637) centre (8.6297, -132.637) ccw
  line L133 (8.6297, -132.137) -> (14.6297, -132.137)
  arc A135 (15.1297, -132.637) -> (14.6297, -132.137) centre (14.6297, -132.637) ccw
  line L134 (15.1297, -132.637) -> (15.1297, -146.637)
  arc A136 (14.6297, -147.137) -> (15.1297, -146.637) centre (14.6297, -146.637) ccw
  line L135 (14.6297, -147.137) -> (8.6297, -147.137)
  arc A137 (35.2668, 194.5943) -> (34.7668, 195.0943) centre (34.7667, 194.5943) ccw
  line L136 (35.2668, 194.5943) -> (35.2668, 181.5943)
  arc A138 (34.7667, 181.0943) -> (35.2668, 181.5943) centre (34.7667, 181.5943) ccw
  line L137 (34.7667, 181.0943) -> (21.7667, 181.0943)
  arc A139 (21.2668, 181.5943) -> (21.7667, 181.0943) centre (21.7668, 181.5943) ccw
  line L138 (21.2668, 181.5943) -> (21.2667, 194.5943)
  arc A140 (21.7668, 195.0943) -> (21.2667, 194.5943) centre (21.7667, 194.5943) ccw
  line L139 (21.7668, 195.0943) -> (34.7668, 195.0943)
  line L140 (-2.8333, -110.2057) -> (-2.8333, -123.2057)
  arc A141 (-3.3333, -123.7057) -> (-2.8333, -123.2057) centre (-3.3333, -123.2057) ccw
  line L141 (-3.3333, -123.7057) -> (-16.3333, -123.7057)
  arc A142 (-16.8333, -123.2057) -> (-16.3333, -123.7057) centre (-16.3333, -123.2057) ccw
  line L142 (-16.8333, -123.2057) -> (-16.8333, -110.2057)
  arc A143 (-16.3333, -109.7057) -> (-16.8333, -110.2057) centre (-16.3333, -110.2057) ccw
  line L143 (-16.3333, -109.7057) -> (-3.3333, -109.7057)
  arc A144 (-2.8333, -110.2057) -> (-3.3333, -109.7057) centre (-3.3333, -110.2057) ccw
  arc A145 (-21.8833, 70.7693) -> (-22.3833, 71.2693) centre (-22.3833, 70.7693) ccw
  line L144 (-21.8833, 70.7693) -> (-21.8833, 57.7693)
  arc A146 (-22.3833, 57.2693) -> (-21.8833, 57.7693) centre (-22.3833, 57.7693) ccw
  line L145 (-22.3833, 57.2693) -> (-35.3833, 57.2693)
  arc A147 (-35.8833, 57.7693) -> (-35.3833, 57.2693) centre (-35.3833, 57.7693) ccw
  line L146 (-35.8833, 57.7693) -> (-35.8833, 70.7693)
  arc A148 (-35.3833, 71.2693) -> (-35.8833, 70.7693) centre (-35.3833, 70.7693) ccw
  line L147 (-35.3833, 71.2693) -> (-22.3833, 71.2693)
  arc A149 (-16.8333, 29.1943) -> (-16.3333, 28.6943) centre (-16.3333, 29.1943) ccw
  line L148 (-16.8333, 29.1943) -> (-16.8333, 42.1943)
  arc A150 (-16.3333, 42.6943) -> (-16.8333, 42.1943) centre (-16.3333, 42.1943) ccw
  line L149 (-16.3333, 42.6943) -> (-3.3333, 42.6943)
  arc A151 (-2.8333, 42.1943) -> (-3.3333, 42.6943) centre (-3.3333, 42.1943) ccw
  line L150 (-2.8333, 42.1943) -> (-2.8333, 29.1943)
  arc A152 (-3.3333, 28.6943) -> (-2.8333, 29.1943) centre (-3.3333, 29.1943) ccw
  line L151 (-3.3333, 28.6943) -> (-16.3333, 28.6943)
  arc A153 (-2.8333, 175.5443) -> (-3.3332, 176.0443) centre (-3.3332, 175.5443) ccw
  line L152 (-2.8333, 175.5443) -> (-2.8332, 162.5443)
  arc A154 (-3.3332, 162.0443) -> (-2.8332, 162.5443) centre (-3.3333, 162.5443) ccw
  line L153 (-3.3332, 162.0443) -> (-16.3333, 162.0443)
  arc A155 (-16.8333, 162.5443) -> (-16.3333, 162.0443) centre (-16.3333, 162.5443) ccw
  line L154 (-16.8333, 162.5443) -> (-16.8332, 175.5443)
  arc A156 (-16.3333, 176.0443) -> (-16.8333, 175.5443) centre (-16.3333, 175.5443) ccw
  line L155 (-16.3333, 176.0443) -> (-3.3332, 176.0443)
  arc A157 (-35.3833, 52.2193) -> (-35.8833, 51.7193) centre (-35.3833, 51.7193) ccw
  line L156 (-35.3833, 52.2193) -> (-22.3833, 52.2193)
  arc A158 (-21.8833, 51.7193) -> (-22.3833, 52.2193) centre (-22.3833, 51.7193) ccw
  line L157 (-21.8833, 51.7193) -> (-21.8833, 38.7193)
  arc A159 (-22.3833, 38.2193) -> (-21.8833, 38.7193) centre (-22.3833, 38.7193) ccw
  line L158 (-22.3833, 38.2193) -> (-35.3833, 38.2193)